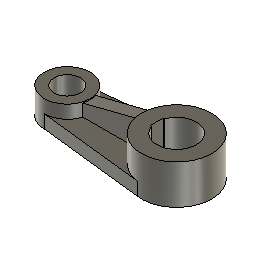
practice 3 (Autodesk Fusion 360 design; units mm, degrees)
part number: 2026-05-21-17-25-35-402
Autodesk Fusion 360 part; units mm, degrees
sketch "Sketch1" plane through (0, 0, 0) normal (0, 0, 1) x (1, 0, 0)
  circle A0 centre (-63.0355, 0) radius 12
  circle A1 centre (-63.0355, 0) radius 21
  circle A2 centre (36.9645, 0) radius 32
  line L0 (-63.0355, 21) -> (33.4028, 31.8012)
  line L1 (-63.0355, -21) -> (33.4028, -31.8012)
  line L2 (18.7234, 6) -> (19.994, 6)
  line L3 (19.994, -6) -> (18.7234, -6)
  line L4 (18.7234, -6) -> (18.7234, 6)
  arc A3 (19.994, -6) -> (19.994, 6) centre (36.9645, 0) ccw
  dimension "d1" = 24
  dimension "d2" = 42
  dimension "d3" = 100
  dimension "d4" = 36
  dimension "d5" = 64
  dimension "d6" = 12
  constraint concentric A0 A1
  constraint concentric A2 A3
  constraint coincident A1 L0.start
  constraint coincident A1 L1.start
  constraint coincident A2 L0.end
  constraint coincident A2 L1.end
  constraint tangent A2 L1
  constraint tangent A2 L0
  constraint horizontal L2
  constraint horizontal L3
  constraint vertical L4
  measures "d1" diameter of A0
  measures "d2" diameter of A1
  measures "d3" distance of A0.centre A2.centre
  measures "d4" diameter of A3
  measures "d5" diameter of A2
  measures "d6" distance of L2.start L3.end
extrude "Extrude1" add sketch "Sketch1" along normal blind 24 contours A1 makes body 1
extrude "Extrude2" add sketch "Sketch1" along normal blind 36 separate body contours A2 makes body 2
extrude "Extrude3" add sketch "Sketch1" along normal blind 12 contours A1 A2 L0 L1 bodies 1 2
sketch "Sketch3" plane through (0, 0, 0) normal (1, 0, 0) x (0, 1, 0)
sketch "Sketch4" plane through (0, 0, 0) normal (0, 1, 0) x (1, 0, 0)
  line L0 (-43, -23) -> (5.9701, -35.4511)
rib "Rib1" add thickness 12 on both sides direction (0.246418, 0, -0.969164) up to next extending the curves path "Sketch4" along L0 bodies 1
